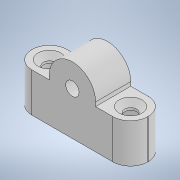
# Autodesk Inventor part: Крышка стойки подшипника 3мм
Saved by Autodesk Inventor 2020 (Build 240168000, 168)
## iProperties
Created: 2021-05-10
Part Number: Крышка стойки подшипника 3мм
Material: Типовые
Document SubType Name: Modeling
Designer: Антон
Density: 1 g/cm^3
Appearance: По умолчанию
Author: Антон
Autodesk Inventor part; units mm, degrees
ref_plane "YZ Plane" through (0, 0, 0) normal (1, 0, 0) x (0, 1, 0)
ref_plane "XZ Plane" through (0, 0, 0) normal (0, 1, 0) x (-1, 0, 0)
ref_plane "XY Plane" through (0, 0, 0) normal (0, 0, 1) x (1, 0, 0)
sketch "Эскиз1" plane through (0, 0, 0) normal (0, 0, 1) x (1, 0, 0)
  circle A0 centre (0, 0) radius 4.05
  line L0 (-6.05, -6.05) -> (6.05, -6.05)
  line L1 (6.05, -6.05) -> (6.05, 6.05)
  line L2 (6.05, 6.05) -> (-6.05, 6.05)
  line L3 (-6.05, 6.05) -> (-6.05, -6.05)
  line L4 (-6.05, -6.05) -> (6.05, 6.05) construction
  line L5 (6.05, -6.05) -> (-6.05, 6.05) construction
  line L6 (0, 4.05) -> (0, 6.05)
  line L7 (-4.05, 0) -> (-6.05, 0)
  line L8 (-15.15, -1.05) -> (0, -1.05)
  line L9 (0, -1.05) -> (0, -3.05)
  line L10 (0, -3.05) -> (-15.15, -3.05)
  line L11 (-15.15, -3.05) -> (-15.15, -1.05)
  line L12 (-4.05, 0) -> (4.05, 0)
  line L13 (4.05, 0) -> (4.05, -3.05)
  line L14 (4.05, -3.05) -> (-4.05, -3.05)
  line L15 (-4.05, -3.05) -> (-4.05, 0)
  line L16 (4.05, -3.05) -> (6.05, -3.05)
  line L17 (6.05, -3.05) -> (6.05, 0)
  line L18 (6.05, 0) -> (4.05, 0)
  line L19 (4.05, 0) -> (4.05, -3.05)
  point P0 (0, -2.05)
  point P1 (0, -6.05)
  point P2 (-6.05, -1.05)
  point P3 (-2.6646, -3.05)
  point P4 (-4.05, -3.05)
  point P5 (2.6646, -3.05)
  point P6 (-6.05, -3.05)
  point P7 (-4.05, -1.05)
  point P8 (-3.9115, -1.05)
  point P9 (-2.6646, -3.05)
  dimension "d0" = 8.1
  dimension "d1" = 2
  dimension "d2" = 2
  dimension "d3" = 9.1
  dimension "d4" = 2
  dimension "d5" = 3
  constraints: 40 end point, 8 parallel, 7 midpoint, 6 perpendicular, 4 horizontal, 3 point on circle, 1 centre point, 1 coincident, 1 point on line, 1 vertical alignment
  measures "d0" diameter of A0
  measures "d1" distance of L6.start L6.end
  measures "d2" distance of L7.start L7.end
  measures "d3" distance between parallel lines of L3 L11
  measures "d4" distance between parallel lines of L10 L8
  measures "d5" distance between parallel lines of L0 L10
extrude "Выдавливание1" add sketch "Эскиз1" along normal blind 1.6 contours A0 L7 L3 L2 L6 | L15 L8 L3 L7 | L15 L10 L3 L8 | L3 L10 L11 L8
sketch "Эскиз2" plane through (0, 0, 1.6) normal (0, 0, 1) x (1, 0, 0)
  line L0 (-6.05, -1.05) -> (-15.15, -1.05) projected
  line L1 (-15.15, -1.05) -> (-15.15, -3.05) projected
  line L2 (-15.15, -3.05) -> (-4.05, -3.05) projected
  line L3 (-4.05, -3.05) -> (-4.05, 0) projected
  arc A0 (0, 4.05) -> (-4.05, 0) centre (0, 0) ccw projected
  line L4 (0, 4.05) -> (0, 6.05) projected
  line L5 (0, 6.05) -> (-6.05, 6.05) projected
  line L6 (-6.05, 6.05) -> (-6.05, -1.05) projected
  line L7 (0, 4.05) -> (-4.05, 4.05)
  line L8 (-4.05, 4.05) -> (-4.05, -3.05)
  line L9 (-4.05, -3.05) -> (0, -3.05)
  line L10 (0, -3.05) -> (0, 4.05)
  constraints: 8 end point, 2 parallel, 1 horizontal, 1 perpendicular
extrude "Выдавливание2" add sketch "Эскиз2" along normal blind 3
mirror "Зеркальное отражение1" about plane through (-9.6, -2.05, 0) normal (0, 0, -1)
sketch "Эскиз4" plane through (-15.15, -1.05, 4.6) normal (0, 1, 0) x (1, 0, 0)
  line L0 (0, 0) -> (0, 9.2) projected
  line L1 (0, 4.6) -> (9.1, 4.6)
  line L2 (9.1, 9.2) -> (9.1, 0) projected
  point P0 (15.15, 4.6)
  point P1 (4.55, 4.6)
  constraints: 3 midpoint, 2 end point, 1 perpendicular
hole "Отверстие2" at (-10.6, -1.05, 0) direction (0, -1, 0) diameter 3.2 end through all countersink diameter 6 countersink angle 90
mirror "Зеркальное отражение2" about plane through (0, 4.05, 0) normal (1, 0, 0)
sketch "Эскиз3" plane through (0, 0, 4.6) normal (0, 0, 1) x (1, 0, 0)
  arc A0 (2.6646, -3.05) -> (4.05, 0) centre (0, 0) ccw projected
  arc A1 (2.6646, -3.05) -> (4.05, 0) centre (0, 0) ccw projected
hole "Отверстие1" at (0, 0, 4.6) direction (0, 0, -1) diameter 3.5 end through all
fillet "Сопряжение1" radius 6.05 2 edges at (-6.05, 6.05, 0) (6.05, 6.05, 0)
sketch "Эскиз7" plane through (-15.15, -3.05, -4.6) normal (0, -1, 0) x (1, 0, 0)
  line L0 (30.3, 0) -> (0, 0) projected
  line L1 (0, 9.2) -> (30.3, 9.2) projected
  line L2 (13.4, 9.2) -> (16.9, 9.2) projected
  line L3 (15.15, 9.2) -> (15.15, 0)
  line L4 (28.3, 2) -> (2, 2)
  line L5 (2, 2) -> (2, 7.2)
  line L6 (2, 7.2) -> (28.3, 7.2)
  line L7 (28.3, 7.2) -> (28.3, 2)
  line L8 (28.3, 2) -> (2, 7.2) construction
  line L9 (2, 2) -> (28.3, 7.2) construction
  line L10 (0, 0) -> (0, 9.2) projected
  line L11 (30.3, 0) -> (30.3, 9.2) projected
  point P0 (15.15, 4.6)
  dimension "d29" = 2
  dimension "d30" = 2
  constraints: 14 end point, 4 midpoint, 2 parallel, 1 horizontal, 1 perpendicular
  measures "d29" distance between parallel lines of L10 L5
  measures "d30" distance between parallel lines of L1 L6
extrude "Выдавливание4" add sketch "Эскиз7" along normal blind 8.25 contours L0 L3 L4 L7 L6 L1 L11 | L0 L10 L1 L3 L6 L5 L4
fillet "Сопряжение2" radius 4.55 4 edges at (15.15, -6.175, -4.6) (15.15, -6.175, 4.6) (-15.15, -6.175, -4.6) (-15.15, -6.175, 4.6)
fillet "Сопряжение3" radius 2.55 4 edges at (13.15, -7.175, -2.6) (13.15, -7.175, 2.6) (-13.15, -7.175, 2.6) (-13.15, -7.175, -2.6)
